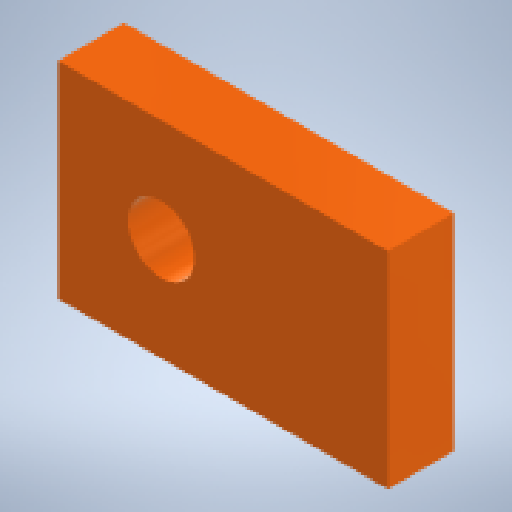
# Autodesk Inventor part: BoltRelease
Saved by Autodesk Inventor 2025.2 (Build 292293000, 293)
## iProperties
Created: 2025-03-16
Part Number: BoltRelease
Material: ABS Plastic
Document SubType Name: Modeling
Designer: baolo
Density: 1.06 g/cm^3
Appearance: Smooth - Light Orange
Author: baolo
Autodesk Inventor part; units mm, degrees
ref_plane "YZ Plane" through (0, 0, 0) normal (1, 0, 0) x (0, 1, 0)
ref_plane "XZ Plane" through (0, 0, 0) normal (0, 1, 0) x (-1, 0, 0)
ref_plane "XY Plane" through (0, 0, 0) normal (0, 0, 1) x (1, 0, 0)
sketch "Sketch1" plane through (0, 0, 0) normal (0, 0, 1) x (1, 0, 0)
  line L0 (-12.5, 12.5) -> (12.5, 12.5)
  line L1 (27.5, 12.5) -> (27.5, -12.5)
  line L2 (12.5, -12.5) -> (-12.5, -12.5)
  line L3 (-12.5, -12.5) -> (-12.5, 12.5)
  line L4 (-12.5, 12.5) -> (12.5, -12.5) construction
  line L5 (12.5, 12.5) -> (-12.5, -12.5) construction
  line L6 (12.5, 12.5) -> (12.5, -12.5) construction
  line L7 (12.5, 12.5) -> (27.5, 12.5)
  line L8 (12.5, -12.5) -> (27.5, -12.5)
  point P0 (0, 0)
  point P1 (0, 0)
  dimension "d0" = 25
  dimension "d1" = 15
  constraints: 18 end point, 3 horizontal, 3 perpendicular, 2 parallel, 1 coincident, 1 midpoint, 1 vertical
  measures "d0" distance between parallel lines of L6 L3
  measures "d1" distance between parallel lines of L6 L1
extrude "Extrusion1" add sketch "Sketch1" along normal mid plane 8
sketch "Sketch2" plane through (0, 0, 4) normal (0, 0, 1) x (1, 0, 0)
  point P0 (0, 0)
hole "Hole1" at (0, 0, 4) direction (0, 0, -1) diameter 8.1 end through all
body "Solid1"
